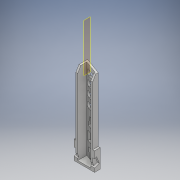
# Autodesk Inventor part: k2_t
Saved by Autodesk Inventor 2017 (Build 210142000, 142)
## iProperties
Created: 2017-02-09
Part Number: k2_t
Material: Generic
Document SubType Name: Modeling
Designer: herman
Density: 1 g/cm^3
Appearance: Default
Author: herman
Autodesk Inventor part; units mm, degrees
ref_plane "YZ Plane" through (0, 0, 0) normal (1, 0, 0) x (0, 1, 0)
ref_plane "XZ Plane" through (0, 0, 0) normal (0, 1, 0) x (-1, 0, 0)
ref_plane "XY Plane" through (0, 0, 0) normal (0, 0, 1) x (1, 0, 0)
sketch "Sketch1" plane through (0, 0, 0) normal (0, 0, 1) x (1, 0, 0)
  line L0 (-8.4365, 10.4464) -> (-8.4365, -8.3808)
  line L1 (-8.4365, -8.3808) -> (18.5635, -8.3808)
  line L2 (18.5635, -8.3808) -> (18.5635, 0.6192)
  line L3 (18.5635, 0.6192) -> (-8.4365, 10.4464)
  point P0 (0, 0)
  dimension "d0" = 9
  dimension "d2" = 110
  dimension "d30" = 27
  constraints: 8 end point, 2 perpendicular, 1 vertical
  measures "d0" distance of L1.end L2.end
  measures "d2" angle of L3 L2
  measures "d30" distance of L0.end L1.end
extrude "Extrusion1" add sketch "Sketch1" along normal blind 200
sketch "Sketch2" plane through (-8.4365, 10.4464, 200) normal (0.3420201, 0.9396926, 0) x (0.9396926, -0.3420201, 0)
  line L0 (7.4677, 159.9801) -> (21.4677, 159.9801)
  line L1 (21.4677, 159.9801) -> (21.4677, 173.9801)
  line L2 (21.4677, 173.9801) -> (7.4677, 173.9801)
  line L3 (7.4677, 173.9801) -> (7.4677, 159.9801)
  line L4 (0, 200) -> (0, 0) projected
  line L5 (28.7328, 200) -> (0, 200) projected
  line L6 (28.7328, 200) -> (28.7328, 0) projected
  line L7 (21.4677, 166.9801) -> (93.4677, 166.9801) construction
  line L8 (23.9211, 148.3451) -> (93.4677, 166.9801) construction
  line L9 (12.2098, 137.9602) -> (25.7328, 141.5836)
  line L10 (25.7328, 141.5836) -> (22.1093, 155.1066)
  line L11 (22.1093, 155.1066) -> (8.5864, 151.4831)
  line L12 (8.5864, 151.4831) -> (12.2098, 137.9602)
  line L13 (8.5864, 182.477) -> (22.1093, 178.8536)
  line L14 (22.1093, 178.8536) -> (25.7328, 192.3765)
  line L15 (25.7328, 192.3765) -> (12.2098, 196)
  line L16 (12.2098, 196) -> (8.5864, 182.477)
  point P0 (11.5006, 200)
  point P1 (23.9211, 185.6151)
  dimension "d5" = 14
  dimension "d6" = 14
  dimension "d9" = 72
  dimension "d12" = 15
  dimension "d16" = 15
  dimension "d19" = 4
  dimension "d46" = 3
  constraints: 28 end point, 2 horizontal, 2 parallel, 1 coincident, 1 midpoint, 1 perpendicular, 21 other
  measures "d5" distance of L1.end L2.end
  measures "d6" distance of L0.end L1.end
  measures "d9" distance of L7.start L7.end
  measures "d19" distance from line of L5 L15.end
  measures "d46" distance from line of L6 L9.end
sketch "Sketch3" plane through (18.5635, -8.3808, 0) normal (1, 0, 0) x (0, 0, -1)
  line L0 (0, 9) -> (-200, 9) projected
  line L1 (0, 9) -> (-30, 9)
  line L2 (-30, 9) -> (-30, 0)
  line L3 (0, 0) -> (0, 9)
  line L4 (0, 9) -> (0, 18.8272) projected
  line L5 (0, 9) -> (0, 0)
  line L6 (0, 0) -> (-6.123, 0)
  line L7 (-18.8931, 0) -> (-30, 0)
  line L8 (0, 0) -> (-200, 0) projected
  line L9 (-18.8931, 0) -> (-20.1355, 3.4133)
  line L10 (-20.1355, 3.4133) -> (-8.8592, 7.5175)
  line L11 (-8.8592, 7.5175) -> (-6.123, 0)
  point P0 (0, 8.3808)
  dimension "d26" = 30
  dimension "d52" = 12
  dimension "d53" = 110
  dimension "d60" = 8
  constraints: 18 end point, 4 perpendicular, 2 horizontal, 1 parallel, 1 point on line
  measures "d26" distance of L0.start L1.end
  measures "d52" distance of L9.end L10.end
  measures "d53" angle of L11 L6
  measures "d60" distance of L6.end L10.end
ref_plane "Work Plane1" through (5.0635, -8.3808, 200) normal (1, 0, 0) x (0, 0, -1)
thicken "Thicken1" operation intersect thickness 3 both sides no extend neighbours no toward (-1, 0, 0) faces at (18.5635, -5.3808, 66.6667) (9.5635, 3.895, 66.6667) (0.5635, 0.895, 0) (-8.4365, 4.1707, 66.6667) (0.5635, 0.895, 200)
extrude "Extrusion6" add sketch "Sketch3" along normal blind 3 contours L3 L6 L11 L10 L9 L7 L2 L0
mirror "Mirror2" about plane through (5.0635, -8.3808, 200) normal (1, 0, 0) of "Extrusion6"
extrude "Extrusion7" cut sketch "Sketch2" against normal up to next
sketch "Sketch5" plane through (18.5635, -8.3808, 18.8931) normal (1, 0, 0) x (0, 0, -1)
  line L0 (12.7701, 0) -> (0, 0) projected
  line L1 (12.7701, 0) -> (10.034, 7.5175) projected
  line L2 (12.0861, 1.8794) -> (6.9225, 0)
  line L3 (12.0861, 1.8794) -> (12.7701, 0)
  line L4 (6.9225, 0) -> (12.7701, 0)
  line L5 (15.8931, 0) -> (-178.1069, 0) projected
  point P0 (18.8931, 8.3808)
  point P1 (-56.5302, 0)
  dimension "d57" = 2
  constraints: 6 end point, 2 collinear, 2 point on line, 1 perpendicular
  measures "d57" distance of L0.start L2.start
extrude "Extrusion8" cut sketch "Sketch5" against normal through all
sketch "Sketch7" plane through (-8.4365, -8.3808, 200) normal (-1, 0, 0) x (0, 0, 1)
  line L0 (-170, 0) -> (0, 0) projected
  line L1 (-200, 18.8272) -> (0, 18.8272) projected
  line L2 (-75.8499, 0) -> (-67.1897, 5)
  line L3 (-67.1897, 5) -> (-67.1897, 18.8272)
  line L4 (-67.1897, 18.8272) -> (0, 18.8272)
  line L5 (0, 9) -> (0, 18.8272) projected
  line L6 (0, 18.8272) -> (0, 0)
  line L7 (0, 0) -> (-75.8499, 0)
  line L8 (-170, 0) -> (-181.1069, 0) projected
  point P0 (-200, 8.3808)
  dimension "d77" = 10
  dimension "d78" = 105.257
  dimension "d79" = 150
  constraints: 10 end point, 3 collinear, 2 point on line, 1 perpendicular
  measures "d77" distance of L2.start L2.end
  measures "d78" distance of L2.start L8.end
  measures "d79" angle of L0 L2
extrude "Extrusion10" cut sketch "Sketch7" against normal through all
sketch "Sketch8" plane through (18.5635, 0.6192, 30) normal (0.3420201, 0.9396926, 0) x (0.9396926, -0.3420201, 0)
  line L0 (-24.4484, 27) -> (-24.4484, -102.8103) construction
  line L1 (-19.4744, -94.1501) -> (-19.4744, 18.0294) projected
  line L2 (-9.1831, -91.3103) -> (-19.1831, -91.3103) construction
  line L3 (-2.1006, -102.8103) -> (-24.4484, -102.8103) projected
  line L4 (-9.1831, -86.8103) -> (-19.1831, -86.8103)
  line L5 (-19.1831, -95.8103) -> (-9.1831, -95.8103)
  arc A0 (-9.1831, -95.8103) -> (-9.1831, -86.8103) centre (-9.1831, -91.3103) ccw
  arc A1 (-19.1831, -86.8103) -> (-19.1831, -95.8103) centre (-19.1831, -91.3103) ccw
  point P0 (-17.2322, 30)
  point P1 (-14.1831, -91.3103)
  point P2 (-18.4744, -93.1501)
  point P3 (-17.4744, -92.1501)
  point P4 (-16.4744, -91.1501)
  dimension "d85" = 9
  dimension "d89" = 10
  dimension "d93" = 7
  constraints: 8 end point, 4 point on circle, 4 tangent, 2 centre point, 2 parallel, 1 midpoint
  measures "d85" diameter of A1
  measures "d89" distance of L2.start L2.end
  measures "d93" distance between parallel lines of L5 L3
extrude "Extrusion11" cut sketch "Sketch8" against normal up to next
pattern_linear "Rectangular Pattern1" count 4 spacing 15 along (0, 0, -1) of "Extrusion11"
body "Solid1"
